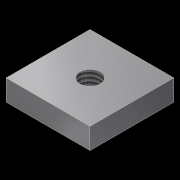
# Autodesk Inventor part: Part1
Saved by Autodesk Inventor 2021.1 (Build 251245000, 245)
## iProperties
Created: 2020-08-29
Part Number: Part1
Material: A5052
Document SubType Name: Modeling
Designer: Hashimoto
Mass: 4.35648 g
Surface Area: 12 cm^2
Volume: 1.6073 cm^3
Density: 2.71043 g/cm^3
Appearance: アルミニウム - つや出し
Author: Hashimoto
Autodesk Inventor part; units mm, degrees
ref_plane "YZ Plane" through (0, 0, 0) normal (1, 0, 0) x (0, 1, 0)
ref_plane "XZ Plane" through (0, 0, 0) normal (0, 1, 0) x (-1, 0, 0)
ref_plane "XY Plane" through (0, 0, 0) normal (0, 0, 1) x (1, 0, 0)
sketch "スケッチ22" plane through (0, 0, 0) normal (0, 0, 1) x (1, 0, 0)
  line L0 (-10, 10) -> (10, 10)
  line L1 (10, 10) -> (10, -10)
  line L2 (10, -10) -> (-10, -10)
  line L3 (-10, -10) -> (-10, 10)
  line L4 (-10, 10) -> (10, -10) construction
  line L5 (10, 10) -> (-10, -10) construction
  point P0 (0, 0)
  dimension "d144" = 20
  dimension "d145" = 20
  constraints: 12 end point, 2 midpoint, 2 parallel, 1 horizontal, 1 perpendicular
  measures "d144" distance of L1.end L2.end
  measures "d145" distance of L0.end L1.end
extrude "押し出し14" add sketch "スケッチ22" along normal blind 5
sketch "スケッチ24" plane through (0, 0, 5) normal (0, 0, 1) x (1, 0, 0)
  point P0 (0, 0)
  point P1 (0, 0)
  constraints: 1 coincident
hole "穴10" at (0, 0, 5) direction (0, 0, -1) diameter 10 end through all
